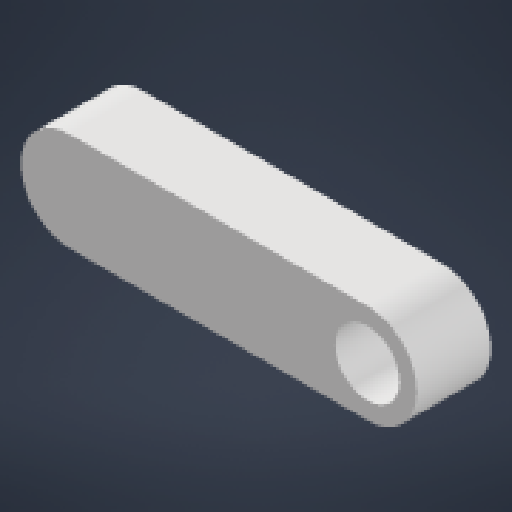
# Autodesk Inventor part: Stands
Saved by Autodesk Inventor 2024.3 (Build 283343000, 343)
## iProperties
Created: 2024-12-16
Part Number: Stands
Material: Generic
Document SubType Name: Modeling
Designer: micha
Density: 1 g/cm^3
Appearance: Default
Author: micha
Autodesk Inventor part; units mm, degrees
ref_plane "YZ Plane" through (0, 0, 0) normal (1, 0, 0) x (0, 1, 0)
ref_plane "XZ Plane" through (0, 0, 0) normal (0, 1, 0) x (-1, 0, 0)
ref_plane "XY Plane" through (0, 0, 0) normal (0, 0, 1) x (1, 0, 0)
sketch "Sketch1" plane through (0, 0, 0) normal (0, 0, 1) x (1, 0, 0)
  circle A0 centre (0, 0) radius 2.0701
  line L0 (0, 0) -> (-19.05, 0) construction
  line L1 (0, 4.7625) -> (-19.05, 4.7625)
  line L2 (-19.05, -4.7625) -> (0, -4.7625)
  arc A1 (0, -4.7625) -> (0, 4.7625) centre (0, 0) ccw
  arc A2 (-19.05, 4.7625) -> (-19.05, -4.7625) centre (-19.05, 0) ccw
  point P0 (-9.525, 0)
  dimension "d0" = 4.1402
  dimension "d2" = 19.05
  dimension "d3" = 9.525
  constraints: 8 end point, 4 point on circle, 4 tangent, 3 centre point, 1 coincident, 1 horizontal, 1 midpoint, 1 parallel
  measures "d0" diameter of A0
  measures "d2" distance of L0.start L0.end
  measures "d3" diameter of A2
extrude "Extrusion1" add sketch "Sketch1" along normal blind 4.7625
fillet "Fillet1" radius 1.5875 4 edges at (4.7625, 0, 4.7625) (-9.525, 4.7625, 4.7625) (-23.8125, 0, 4.7625) (-9.525, -4.7625, 4.7625)
body "Solid1"
